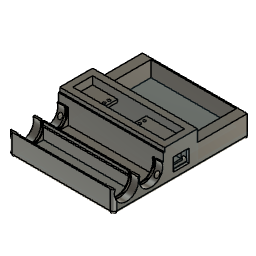
servo holder v10 (Autodesk Fusion 360 design; units mm, degrees)
Autodesk Fusion 360 part; units mm, degrees
sketch "Sketch1" plane through (0, 0, 0) normal (0, 0, 1) x (1, 0, 0)
  line L0 (35, 7.5) -> (-35, 7.5)
  line L1 (-35, 7.5) -> (-35, -7.5)
  line L2 (-35, -7.5) -> (35, -7.5)
  line L3 (35, -7.5) -> (35, 7.5)
  line L4 (35, 7.5) -> (-35, -7.5) construction
  line L5 (-35, 7.5) -> (35, -7.5) construction
  dimension "d1" = 70
  dimension "d2" = 15
  constraint horizontal L0
  constraint perpendicular L0 L1
  constraint parallel L0 L2
  constraint parallel L1 L3
  constraint coincident L4 origin
  constraint coincident L5 origin
  measures "d1" distance of L1.end L2.end
  measures "d2" distance of L0.end L1.end
extrude "Extrude1" add sketch "Sketch1" along normal blind 5
sketch "Sketch2" plane through (0, 0, 5) normal (0, 0, 1) x (-1, 0, 0)
  line L0 (-35, 7.5) -> (-35, -7.5)
  line L1 (-35, -7.5) -> (35, -7.5)
  line L2 (35, -7.5) -> (35, 7.5)
  line L3 (35, 7.5) -> (-35, 7.5)
sketch "Sketch3" plane through (0, 0, 0) normal (0, 0, -1) x (1, 0, 0)
  line L0 (35, -7.5) -> (35, 7.5)
  line L1 (35, 7.5) -> (-35, 7.5)
  line L2 (-35, 7.5) -> (-35, -7.5)
  line L3 (-35, -7.5) -> (35, -7.5)
  line L4 (35, 7.5) -> (40, 7.5)
  line L5 (40, 7.5) -> (40, -7.5)
  line L6 (40, -7.5) -> (35, -7.5)
  line L7 (35, -7.5) -> (35, 7.5)
  line L8 (-35, 7.5) -> (-40, 7.5)
  line L9 (-40, 7.5) -> (-40, -7.5)
  line L10 (-40, -7.5) -> (-35, -7.5)
  line L11 (-35, -7.5) -> (-35, 7.5)
  dimension "d9" = 5
  dimension "d10" = 15
  dimension "d11" = 5
  dimension "d12" = 15
  constraint horizontal L4
  constraint vertical L5
  constraint horizontal L6
  constraint vertical L7
  constraint coincident L0.end L1.start
  constraint horizontal L8
  constraint vertical L9
  constraint horizontal L10
  constraint vertical L11
  constraint coincident L1.end L2.start
  measures "d9" distance of L0.end L4.end
  measures "d10" distance of L0.end L0.start
  measures "d11" distance of L1.end L8.end
  measures "d12" distance of L1.end L2.end
extrude "Extrude2" add sketch "Sketch3" against normal blind 26 contours L0 L4 L5 L6 L7 | L2 L8 L9 L10 L11
sketch "Sketch4" plane through (0, -7.5, 0) normal (0, -1, 0) x (1, 0, 0)
  line L0 (-40, 0) -> (40, 0)
  line L1 (40, 0) -> (40, 26)
  line L2 (40, 26) -> (35, 26)
  line L3 (35, 26) -> (35, 5)
  line L4 (35, 5) -> (-35, 5)
  line L5 (-35, 5) -> (-35, 26)
  line L6 (-35, 26) -> (-40, 26)
  line L7 (-40, 26) -> (-40, 0)
  line L8 (6, 20) -> (35, 20)
  line L9 (35, 20) -> (35, 18)
  line L10 (35, 18) -> (6, 18)
  line L11 (6, 18) -> (6, 20)
  line L12 (-35, 5) -> (35, 5)
  line L13 (-35, 20) -> (-16, 20)
  line L14 (-16, 20) -> (-16, 18)
  line L15 (-16, 18) -> (-35, 18)
  line L16 (-35, 18) -> (-35, 20)
  dimension "d15" = 29
  dimension "d16" = 2
  dimension "d17" = 13
  dimension "d18" = 5
  dimension "d19" = 19
  dimension "d20" = 2
  dimension "d21" = 13
  dimension "d22" = 5
  constraint horizontal L8
  constraint vertical L9
  constraint horizontal L10
  constraint vertical L11
  constraint horizontal L13
  constraint vertical L14
  constraint horizontal L15
  constraint vertical L16
  measures "d15" distance of L8.start L8.end
  measures "d16" distance of L8.start L10.end
  measures "d17" distance of L10 L12
  measures "d18" distance of L1 L9
  measures "d19" distance of L13.start L13.end
  measures "d20" distance of L13.start L15.end
  measures "d21" distance of L12 L15
  measures "d22" distance of L7 L13.start
extrude "Extrude3" add sketch "Sketch4" against normal blind 15 contours L5 L13 L14 L15 L16 | L3 L8 L9 L10 L11
sketch "Sketch5" plane through (0, 0, 20) normal (0, 0, 1) x (-1, 0, 0)
  line L0 (-6, 7.5) -> (-35, 7.5)
  line L1 (-35, 7.5) -> (-35, -7.5)
  line L2 (-35, -7.5) -> (-6, -7.5)
  line L3 (-6, -7.5) -> (-6, 7.5)
  circle A0 centre (-8.54, 3.5) radius 1
  circle A1 centre (-8.54, -3.5) radius 1
  circle A2 centre (-8.54, 0) radius 1
  circle A3 centre (-8.54, 3.5) radius 1
  circle A4 centre (-8.54, 0) radius 1
  circle A5 centre (18.54, 3.5) radius 1
  circle A6 centre (18.54, -3.5) radius 1
  circle A7 centre (18.54, 0) radius 1
  line L4 (16, 7.5) -> (16, -7.5)
  dimension "d25" = 2
  dimension "d36" = 2
  dimension "d44" = 2
  dimension "d45" = 2.54
  dimension "d48" = 3.5
  dimension "d49" = 3.5
  dimension "d50" = 2
  dimension "d53" = 3.5
  dimension "d55" = 2
  dimension "d56" = 2
  dimension "d57" = 2
  dimension "d58" = 3.5
  dimension "d59" = 3.5
  dimension "d60" = 2.54
  measures "d25" diameter of A0
  measures "d36" diameter of A1
  measures "d44" diameter of A2
  measures "d45" distance of L3 A2.centre
  measures "d48" distance of A0.centre A2.centre
  measures "d49" distance of A1.centre A2.centre
  measures "d50" diameter of A3
  measures "d53" distance of A2.centre A0.centre
  measures "d55" diameter of A5
  measures "d56" diameter of A6
  measures "d57" diameter of A7
  measures "d58" distance of A7.centre A5.centre
  measures "d59" distance of A7.centre A6.centre
  measures "d60" distance of A7.centre L4
extrude "Extrude4" cut sketch "Sketch5" against normal blind 2 contours A0 A3 | A1 | A2 A4 | A5 | A6 | A7
sketch "Sketch6" plane through (0, 0, 0) normal (0, 0, -1) x (1, 0, 0)
  line L0 (40, 7.5) -> (-40, 7.5)
  line L1 (-40, 7.5) -> (-40, -7.5)
  line L2 (-40, -7.5) -> (40, -7.5)
  line L3 (40, -7.5) -> (40, 7.5)
  line L4 (-40, 7.5) -> (40, 7.5)
  line L5 (40, 7.5) -> (40, 12.5)
  line L6 (40, 12.5) -> (-40, 12.5)
  line L7 (-40, 12.5) -> (-40, 7.5)
  line L8 (-40, -7.5) -> (40, -7.5)
  line L9 (40, -7.5) -> (40, -12.5)
  line L10 (40, -12.5) -> (-40, -12.5)
  line L11 (-40, -12.5) -> (-40, -7.5)
  dimension "d63" = 80
  dimension "d64" = 5
  dimension "d65" = 80
  dimension "d66" = 5
  constraint horizontal L4
  constraint vertical L5
  constraint horizontal L6
  constraint vertical L7
  constraint coincident L0.end L1.start
  constraint horizontal L8
  constraint vertical L9
  constraint horizontal L10
  constraint vertical L11
  constraint coincident L1.end L2.start
  measures "d63" distance of L0.end L0.start
  measures "d64" distance of L0.end L6.end
  measures "d65" distance of L1.end L2.end
  measures "d66" distance of L1.end L10.end
extrude "Extrude5" add sketch "Sketch6" against normal blind 26 contours L0 L4 L5 L6 L7 | L2 L8 L9 L10 L11
sketch "Sketch7" plane through (0, 0, 5) normal (0, 0, 1) x (1, 0, 0)
  line L0 (-15.5, 7.5) -> (5.5, 7.5)
  line L1 (5.5, 7.5) -> (5.5, 6.1)
  line L2 (5.5, 6.1) -> (-15.5, 6.1)
  line L3 (-15.5, 6.1) -> (-15.5, 7.5)
  line L4 (-15.3542, -7.4527) -> (5.6458, -7.4527)
  line L5 (5.6458, -7.4527) -> (5.6458, -6.0527)
  line L6 (5.6458, -6.0527) -> (-15.3542, -6.0527)
  line L7 (-15.3542, -6.0527) -> (-15.3542, -7.4527)
  dimension "d69" = 21
  dimension "d70" = 1.4
  dimension "d71" = 21
  dimension "d72" = 1.4
  constraint horizontal L0
  constraint vertical L1
  constraint horizontal L2
  constraint vertical L3
  constraint horizontal L4
  constraint vertical L5
  constraint horizontal L6
  constraint vertical L7
  measures "d69" distance of L0.start L0.end
  measures "d70" distance of L0.start L2.end
  measures "d71" distance of L4.start L4.end
  measures "d72" distance of L4.start L6.end
extrude "Extrude6" add sketch "Sketch7" along normal blind 5
sketch "Sketch8" plane through (40, 0, 0) normal (1, 0, 0) x (0, 1, 0)
  line L0 (-12.5, 0) -> (12.5, 0)
  line L1 (12.5, 0) -> (12.5, 26)
  line L2 (12.5, 26) -> (-12.5, 26)
  line L3 (-12.5, 26) -> (-12.5, 0)
  line L4 (-5, 15.5) -> (5, 15.5)
  line L5 (5, 15.5) -> (5, 7.5)
  line L6 (5, 7.5) -> (-5, 7.5)
  line L7 (-5, 7.5) -> (-5, 15.5)
  dimension "d75" = 10
  dimension "d76" = 8
  dimension "d77" = 7.5
  dimension "d78" = 7.5
  constraint horizontal L4
  constraint vertical L5
  constraint horizontal L6
  constraint vertical L7
  measures "d75" distance of L4.start L4.end
  measures "d76" distance of L4.start L6.end
  measures "d77" distance of L1 L5
  measures "d78" distance of L0 L6
extrude "Extrude7" cut sketch "Sketch8" against normal blind 5 contours L4 L5 L6 L7
sketch "Sketch9" plane through (0, 0, 0) normal (0, 0, -1) x (1, 0, 0)
  line L0 (-40, 12.5) -> (-40, -12.5)
  line L1 (-40, -12.5) -> (40, -12.5)
  line L2 (40, -12.5) -> (40, 12.5)
  line L3 (40, 12.5) -> (-40, 12.5)
  line L4 (-40, 12.5) -> (40, 12.5)
  line L5 (40, 12.5) -> (40, 32.5)
  line L6 (40, 32.5) -> (-40, 32.5)
  line L7 (-40, 32.5) -> (-40, 12.5)
  dimension "d81" = 80
  dimension "d82" = 20
  constraint horizontal L4
  constraint vertical L5
  constraint horizontal L6
  constraint vertical L7
  constraint coincident L0.start L3.end
  measures "d81" distance of L0.start L2.end
  measures "d82" distance of L0.start L6.end
extrude "Extrude8" add sketch "Sketch9" against normal blind 5 contours L3 L4 L5 L6 L7
sketch "Sketch10" plane through (0, 0, 5) normal (0, 0, 1) x (-1, 0, 0)
  line L0 (40, 12.5) -> (40, 32.5)
  line L1 (40, 32.5) -> (-40, 32.5)
  line L2 (-40, 32.5) -> (-40, 12.5)
  line L3 (-40, 12.5) -> (40, 12.5)
  line L4 (40, 12.5) -> (-40, 12.5)
  line L5 (-40, 12.5) -> (-40, 13.5)
  line L6 (-40, 13.5) -> (40, 13.5)
  line L7 (40, 13.5) -> (40, 12.5)
  dimension "d85" = 80
  dimension "d86" = 1
  constraint horizontal L4
  constraint vertical L5
  constraint horizontal L6
  constraint vertical L7
  constraint coincident L0.start L3.end
  measures "d85" distance of L0.start L2.end
  measures "d86" distance of L0.start L6.end
extrude "Extrude9" add sketch "Sketch10" along normal blind 18 contours L0 L2 L3 L4 L5 L6 L7
sketch "Sketch11" plane through (0, 0, 5) normal (0, 0, 1) x (-1, 0, 0)
  line L0 (-40, 13.5) -> (40, 13.5)
  line L1 (40, 13.5) -> (40, 32.5)
  line L2 (40, 32.5) -> (-40, 32.5)
  line L3 (-40, 32.5) -> (-40, 13.5)
  line L4 (-40, 13.5) -> (-33.5, 13.5)
  line L5 (-33.5, 13.5) -> (-33.5, 32.5)
  line L6 (-33.5, 32.5) -> (-40, 32.5)
  line L7 (-40, 32.5) -> (-40, 13.5)
  line L8 (40, 13.5) -> (33.5, 13.5)
  line L9 (33.5, 13.5) -> (33.5, 32.5)
  line L10 (33.5, 32.5) -> (40, 32.5)
  line L11 (40, 32.5) -> (40, 13.5)
  dimension "d89" = 6.5
  dimension "d90" = 6.5
  constraint horizontal L4
  constraint vertical L5
  constraint horizontal L6
  constraint vertical L7
  constraint coincident L0.start L3.end
  constraint horizontal L8
  constraint vertical L9
  constraint horizontal L10
  constraint vertical L11
  constraint coincident L0.end L1.start
  measures "d89" distance of L0.start L4.end
  measures "d90" distance of L0.end L8.end
extrude "Extrude10" add sketch "Sketch11" along normal blind 12 contours L0 L2 L3 L4 L5 L6 L7 | L0 L1 L2 L8 L9 L10 L11
sketch "Sketch12" plane through (40, 0, 0) normal (1, 0, 0) x (0, 1, 0)
  line L0 (5, 15.5) -> (5, 7.5)
  line L1 (5, 7.5) -> (-5, 7.5)
  line L2 (-5, 7.5) -> (-5, 15.5)
  line L3 (-5, 15.5) -> (5, 15.5)
  line L4 (-32.5, 0) -> (12.5, 0)
  line L5 (12.5, 0) -> (12.5, 26)
  line L6 (12.5, 26) -> (-12.5, 26)
  line L7 (-12.5, 26) -> (-12.5, 23)
  line L8 (-12.5, 23) -> (-13.5, 23)
  line L9 (-13.5, 23) -> (-13.5, 17)
  line L10 (-13.5, 17) -> (-32.5, 17)
  line L11 (-32.5, 17) -> (-32.5, 0)
  circle A0 centre (-23, 14) radius 9
  dimension "d93" = 18
  dimension "d94" = 14
  dimension "d95" = 9.5
  measures "d93" diameter of A0
  measures "d94" distance of L4 A0.centre
  measures "d95" distance of L11 A0.centre
extrude "Extrude11" cut sketch "Sketch12" against normal blind 80 contours L10 A0 | L10 A0
sketch "Sketch13" plane through (0, 0, 5) normal (0, 0, 1) x (-1, 0, 0)
  line L0 (33.5, 23) -> (33.5, 32.5)
  line L1 (33.5, 32.5) -> (-33.5, 32.5)
  line L2 (-33.5, 32.5) -> (-33.5, 23)
  line L3 (-33.5, 23) -> (-33.5, 13.5)
  line L4 (-33.5, 13.5) -> (33.5, 13.5)
  line L5 (33.5, 13.5) -> (33.5, 23)
  line L6 (33.5, 13.5) -> (32.5, 13.5)
  line L7 (32.5, 13.5) -> (32.5, 32.5)
  line L8 (32.5, 32.5) -> (33.5, 32.5)
  line L9 (33.5, 32.5) -> (33.5, 13.5)
  line L10 (-33.5, 13.5) -> (-32.5, 13.5)
  line L11 (-32.5, 13.5) -> (-32.5, 32.5)
  line L12 (-32.5, 32.5) -> (-33.5, 32.5)
  line L13 (-33.5, 32.5) -> (-33.5, 13.5)
  dimension "d98" = 1
  dimension "d99" = 1
  constraint horizontal L6
  constraint vertical L7
  constraint horizontal L8
  constraint vertical L9
  constraint coincident L4.end L5.start
  constraint horizontal L10
  constraint vertical L11
  constraint horizontal L12
  constraint vertical L13
  constraint coincident L3.end L4.start
  measures "d98" distance of L4.end L6.end
  measures "d99" distance of L3.end L10.end
extrude "Extrude12" add sketch "Sketch13" along normal blind 12 contours L0 L1 L4 L5 L6 L7 L8 L9 | L1 L2 L3 L4 L10 L11 L12 L13
delete_face "DeleteFace1" 1 faces at (33.5, -20.1151, 14.4205)
delete_face "DeleteFace2" 1 faces at (-33.5, -25.1677, 12.4715)
sketch "Sketch14" plane through (0, 0, 5) normal (0, 0, 1) x (-1, 0, 0)
  line L0 (-32.5, 23) -> (-32.5, 13.5)
  line L1 (-32.5, 13.5) -> (32.5, 13.5)
  line L2 (32.5, 13.5) -> (32.5, 23)
  line L3 (32.5, 23) -> (32.5, 32.5)
  line L4 (32.5, 32.5) -> (-32.5, 32.5)
  line L5 (-32.5, 32.5) -> (-32.5, 23)
  line L6 (-33, 13.5) -> (-34.5, 13.5)
  line L7 (-34.5, 13.5) -> (-34.5, 32.5)
  line L8 (-34.5, 32.5) -> (-33, 32.5)
  line L9 (-33, 32.5) -> (-33, 13.5)
  dimension "d102" = 1.5
  dimension "d103" = 19
  dimension "d104" = 0.5
  constraint horizontal L6
  constraint vertical L7
  constraint horizontal L8
  constraint vertical L9
  measures "d102" distance of L6.start L6.end
  measures "d103" distance of L6.start L8.end
  measures "d104" distance of L0 L9
extrude "Extrude13" cut sketch "Sketch14" along normal blind 12 contours L6 L7 L8 L9
sketch "Sketch15" plane through (0, 0, 5) normal (0, 0, 1) x (-1, 0, 0)
  line L0 (-32.5, 23) -> (-32.5, 13.5)
  line L1 (-32.5, 13.5) -> (32.5, 13.5)
  line L2 (32.5, 13.5) -> (32.5, 23)
  line L3 (32.5, 23) -> (32.5, 32.5)
  line L4 (32.5, 32.5) -> (-32.5, 32.5)
  line L5 (-32.5, 32.5) -> (-32.5, 23)
  line L6 (34.5, 13.5004) -> (33, 13.5004)
  line L7 (33, 13.5004) -> (33, 32.5004)
  line L8 (33, 32.5004) -> (34.5, 32.5004)
  line L9 (34.5, 32.5004) -> (34.5, 13.5004)
  dimension "d107" = 1.5
  dimension "d108" = 19
  dimension "d109" = 0.5
  constraint horizontal L6
  constraint vertical L7
  constraint horizontal L8
  constraint vertical L9
  measures "d107" distance of L6.start L6.end
  measures "d108" distance of L6.start L8.end
  measures "d109" distance of L2 L7
extrude "Extrude14" cut sketch "Sketch15" along normal blind 12 contours L6 L7 L8 L9
sketch "Sketch16" plane through (0, 0, 0) normal (0, 0, -1) x (1, 0, 0)
  line L0 (-40, 32.5) -> (-40, -12.5)
  line L1 (-40, -12.5) -> (40, -12.5)
  line L2 (40, -12.5) -> (40, 32.5)
  line L3 (40, 32.5) -> (-40, 32.5)
  line L4 (-40, 32.5) -> (40, 32.5)
  line L5 (40, 32.5) -> (40, 51.5)
  line L6 (40, 51.5) -> (-40, 51.5)
  line L7 (-40, 51.5) -> (-40, 32.5)
  line L8 (40, -12.5) -> (-40, -12.5)
  line L9 (-40, -12.5) -> (-40, -50.5)
  line L10 (-40, -50.5) -> (40, -50.5)
  line L11 (40, -50.5) -> (40, -12.5)
  dimension "d112" = 80
  dimension "d113" = 19
  dimension "d114" = 80
  dimension "d115" = 38
  constraint horizontal L4
  constraint vertical L5
  constraint horizontal L6
  constraint vertical L7
  constraint coincident L0.start L3.end
  constraint horizontal L8
  constraint vertical L9
  constraint horizontal L10
  constraint vertical L11
  constraint coincident L1.end L2.start
  measures "d112" distance of L0.start L2.end
  measures "d113" distance of L0.start L6.end
  measures "d114" distance of L1.end L0.end
  measures "d115" distance of L1.end L10.end
extrude "Extrude15" add sketch "Sketch16" against normal blind 5 contours L3 L4 L5 L6 L7 | L1 L8 L9 L10 L11
sketch "Sketch17" plane through (0, 0, 5) normal (0, 0, 1) x (-1, 0, 0)
  line L0 (33, 32.5) -> (33, 23)
  line L1 (33, 23) -> (33, 13.5004)
  line L2 (33, 13.5004) -> (34.5, 13.5004)
  line L3 (34.5, 13.5004) -> (34.5, 23)
  line L4 (34.5, 23) -> (34.5, 32.5)
  line L5 (34.5, 32.5) -> (40, 32.5)
  line L6 (40, 32.5) -> (40, 51.5)
  line L7 (40, 51.5) -> (-40, 51.5)
  line L8 (-40, 51.5) -> (-40, 32.5)
  line L9 (-40, 32.5) -> (-34.5, 32.5)
  line L10 (-34.5, 32.5) -> (-34.5, 23)
  line L11 (-34.5, 23) -> (-34.5, 13.5)
  line L12 (-34.5, 13.5) -> (-33, 13.5)
  line L13 (-33, 13.5) -> (-33, 23)
  line L14 (-33, 23) -> (-33, 32.5)
  line L15 (-33, 32.5) -> (-32.5, 32.5)
  line L16 (-32.5, 32.5) -> (-32.5, 23)
  line L17 (-32.5, 23) -> (-32.5, 13.5)
  line L18 (-32.5, 13.5) -> (32.5, 13.5)
  line L19 (32.5, 13.5) -> (32.5, 23)
  line L20 (32.5, 23) -> (32.5, 32.5)
  line L21 (32.5, 32.5) -> (33, 32.5)
  line L22 (40, 32.5) -> (32.5, 32.5)
  line L23 (32.5, 32.5) -> (32.5, 51.5)
  line L24 (32.5, 51.5) -> (40, 51.5)
  line L25 (40, 51.5) -> (40, 32.5)
  line L26 (-40, 32.5) -> (-32.5, 32.5)
  line L27 (-32.5, 32.5) -> (-32.5, 51.5)
  line L28 (-32.5, 51.5) -> (-40, 51.5)
  line L29 (-40, 51.5) -> (-40, 32.5)
  dimension "d118" = 7.5
  dimension "d119" = 19
  dimension "d120" = 7.5
  dimension "d121" = 19
  constraint horizontal L22
  constraint vertical L23
  constraint horizontal L24
  constraint vertical L25
  constraint coincident L5.end L6.start
  constraint horizontal L26
  constraint vertical L27
  constraint horizontal L28
  constraint vertical L29
  constraint coincident L8.end L9.start
  measures "d118" distance of L5.end L20.end
  measures "d119" distance of L5.end L6.end
  measures "d120" distance of L8.end L15.end
  measures "d121" distance of L8.end L7.end
extrude "Extrude16" add sketch "Sketch17" along normal blind 12 contours L5 L6 L7 L21 L22 L23 L24 L25 | L7 L8 L9 L15 L26 L27 L28 L29
sketch "Sketch18" plane through (0, 0, 5) normal (0, 0, 1) x (-1, 0, 0)
  line L0 (32.5, 23) -> (32.5, 51.5)
  line L1 (32.5, 51.5) -> (-32.5, 51.5)
  line L2 (-32.5, 51.5) -> (-32.5, 23)
  line L3 (-32.5, 23) -> (-32.5, 13.5)
  line L4 (-32.5, 13.5) -> (32.5, 13.5)
  line L5 (32.5, 13.5) -> (32.5, 23)
  line L6 (-32.5, 31.5206) -> (32.5, 31.5206)
  line L7 (32.5, 31.5206) -> (32.5, 32.5206)
  line L8 (32.5, 32.5206) -> (-32.5, 32.5206)
  line L9 (-32.5, 32.5206) -> (-32.5, 31.5206)
  dimension "d124" = 1
  constraint horizontal L6
  constraint vertical L7
  constraint horizontal L8
  constraint vertical L9
  constraint coincident L2 L6.start
  measures "d124" distance of L6.start L8.end
extrude "Extrude17" add sketch "Sketch18" along normal blind 12 contours L0 L2 L6 L7 L8 L9
sketch "Sketch19" plane through (0, 0, 5) normal (0, 0, 1) x (-1, 0, 0)
  line L0 (-32.5, 32.5206) -> (32.5, 32.5206)
  line L1 (32.5, 32.5206) -> (32.5, 51.5)
  line L2 (32.5, 51.5) -> (-32.5, 51.5)
  line L3 (-32.5, 51.5) -> (-32.5, 32.5206)
sketch "Sketch21" plane through (0, 0, 17) normal (0, 0, 1) x (-1, 0, 0)
  line L0 (33, 31.4853) -> (33, 32.5)
  line L1 (33, 32.5) -> (34.5, 32.5)
  line L2 (34.5, 32.5) -> (34.5, 31.4853)
  line L3 (34.5, 31.4853) -> (40, 31.4853)
  line L4 (40, 31.4853) -> (40, 51.5)
  line L5 (40, 51.5) -> (32.5, 51.5)
  line L6 (32.5, 51.5) -> (32.5, 32.5206)
  line L7 (32.5, 32.5206) -> (-32.5, 32.5206)
  line L8 (-32.5, 32.5206) -> (-32.5, 51.5)
  line L9 (-32.5, 51.5) -> (-40, 51.5)
  line L10 (-40, 51.5) -> (-40, 31.4853)
  line L11 (-40, 31.4853) -> (-34.5, 31.4853)
  line L12 (-34.5, 31.4853) -> (-34.5, 32.5)
  line L13 (-34.5, 32.5) -> (-33, 32.5)
  line L14 (-33, 32.5) -> (-33, 31.4853)
  line L15 (-33, 31.4853) -> (-32.5, 31.4853)
  line L16 (-32.5, 31.4853) -> (-32.5, 31.5206)
  line L17 (-32.5, 31.5206) -> (32.5, 31.5206)
  line L18 (32.5, 31.5206) -> (32.5, 31.4853)
  line L19 (32.5, 31.4853) -> (33, 31.4853)
  line L20 (34.5, 32.5) -> (33, 32.5)
  line L21 (33, 32.5) -> (33, 50.5)
  line L22 (33, 50.5) -> (34.5, 50.5)
  line L23 (34.5, 50.5) -> (34.5, 32.5)
  line L24 (-34.5, 32.5) -> (-33, 32.5)
  line L25 (-33, 32.5) -> (-33, 50.5)
  line L26 (-33, 50.5) -> (-34.5, 50.5)
  line L27 (-34.5, 50.5) -> (-34.5, 32.5)
  line L28 (32.5, 51.5) -> (-32.5, 51.5)
  line L29 (-32.5, 51.5) -> (-32.5, 50.5)
  line L30 (-32.5, 50.5) -> (32.5, 50.5)
  line L31 (32.5, 50.5) -> (32.5, 51.5)
  dimension "d129" = 1.5
  dimension "d130" = 18
  dimension "d131" = 1.5
  dimension "d132" = 18
  dimension "d133" = 65
  dimension "d134" = 1
  constraint horizontal L20
  constraint vertical L21
  constraint horizontal L22
  constraint vertical L23
  constraint coincident L1.end L2.start
  constraint horizontal L24
  constraint vertical L25
  constraint horizontal L26
  constraint vertical L27
  constraint coincident L12.end L13.start
  constraint horizontal L28
  constraint vertical L29
  constraint horizontal L30
  constraint vertical L31
  constraint coincident L5.end L6.start
  measures "d129" distance of L1.end L0.end
  measures "d130" distance of L1.end L22.end
  measures "d131" distance of L12.end L13.end
  measures "d132" distance of L12.end L26.end
  measures "d133" distance of L5.end L8.end
  measures "d134" distance of L5.end L30.end
extrude "Extrude18" cut sketch "Sketch21" against normal blind 12 contours L1 L20 L21 L22 L23 | L13 L24 L25 L26 L27
sketch "Sketch22" plane through (0, 0, 5) normal (0, 0, 1) x (1, 0, 0)
sketch "Sketch23" plane through (0, 0, 5) normal (0, 0, 1) x (1, 0, 0)
sketch "Sketch24" plane through (32.5, 0, 0) normal (-1, 0, 0) x (0, -1, 0)
  line L0 (32.5206, 17) -> (32.5206, 5)
  line L1 (32.5206, 5) -> (51.5, 5)
  line L2 (51.5, 5) -> (51.5, 17)
  line L3 (51.5, 17) -> (32.5206, 17)
  line L4 (51.5, 17) -> (50.5, 17)
  line L5 (50.5, 17) -> (50.5, 5)
  line L6 (50.5, 5) -> (51.5, 5)
  line L7 (51.5, 5) -> (51.5, 17)
  dimension "d137" = 1
  dimension "d138" = 12
  constraint horizontal L4
  constraint vertical L5
  constraint horizontal L6
  constraint vertical L7
  constraint coincident L2.end L3.start
  measures "d137" distance of L2.end L4.end
  measures "d138" distance of L2.end L1.end
extrude "Extrude19" add sketch "Sketch24" along normal blind 65 contours L1 L2 L3 L4 L5 L6 L7
sketch "Sketch25" plane through (40, 0, 0) normal (1, 0, 0) x (0, 1, 0)
  arc A0 (-31.4853, 17) -> (-14.5147, 17) centre (-23, 14) ccw
  line L0 (-31.4853, 17) -> (-51.5, 17)
  line L1 (-51.5, 17) -> (-51.5, 0)
  line L2 (-51.5, 0) -> (50.5, 0)
  line L3 (50.5, 0) -> (50.5, 5)
  line L4 (50.5, 5) -> (12.5, 5)
  line L5 (12.5, 5) -> (12.5, 26)
  line L6 (12.5, 26) -> (-12.5, 26)
  line L7 (-12.5, 26) -> (-12.5, 23)
  line L8 (-12.5, 23) -> (-13.5, 23)
  line L9 (-13.5, 23) -> (-13.5, 17)
  line L10 (-13.5, 17) -> (-14.5147, 17)
  line L11 (5, 15.5) -> (5, 7.5)
  line L12 (5, 7.5) -> (-5, 7.5)
  line L13 (-5, 7.5) -> (-5, 15.5)
  line L14 (-5, 15.5) -> (5, 15.5)
  circle A1 centre (-41.5, 14) radius 9
  dimension "d141" = 18
  dimension "d142" = 14
  dimension "d143" = 10
  measures "d141" diameter of A1
  measures "d142" distance of L2 A1.centre
  measures "d143" distance of L1 A1.centre
extrude "Extrude20" cut sketch "Sketch25" against normal blind 80 contours L0 A1 | L0 A1
fillet "Fillet1" radius 2.5 1 edges at (0, -51.5, 0)
fillet "Fillet2" radius 2.5 3 edges at (-40, 0.75, 0) (-40, -50.7678, 0.7322) (-40, -51.5, 9.75)
fillet "Fillet3" radius 2.5 3 edges at (40, 0.75, 0) (40, -50.7678, 0.7322) (40, -51.5, 9.75)
sketch "Sketch27" plane through (0, 12.5, 0) normal (0, 1, 0) x (-1, 0, 0)
  line L0 (-40, 5) -> (40, 5)
  line L1 (40, 5) -> (40, 26)
  line L2 (40, 26) -> (-40, 26)
  line L3 (-40, 26) -> (-40, 5)
  circle A0 centre (37, 9.75) radius 1.75
  dimension "d155" = 3.5
  dimension "d156" = 3
  dimension "d157" = 4.75
  measures "d155" diameter of A0
  measures "d156" distance of L1 A0.centre
  measures "d157" distance of L0 A0.centre
extrude "Extrude21" cut sketch "Sketch27" along normal blind -30 and the other way blind -10 contours A0
sketch "Sketch28" plane through (0, 12.5, 0) normal (0, 1, 0) x (-1, 0, 0)
  circle A0 centre (37, 9.75) radius 1.75
  line L0 (-40, 5) -> (40, 5)
  line L1 (40, 5) -> (40, 26)
  line L2 (40, 26) -> (-40, 26)
  line L3 (-40, 26) -> (-40, 5)
  circle A1 centre (-37.5, 8.75) radius 1.75
  dimension "d162" = 3.5
  dimension "d163" = 2.5
  dimension "d164" = 3.75
  measures "d162" diameter of A1
  measures "d163" distance of L3 A1.centre
  measures "d164" distance of L0 A1.centre
extrude "Extrude22" cut sketch "Sketch28" against normal blind 30 contours A1
sketch "Sketch29" plane through (40, 0, 0) normal (1, 0, 0) x (0, 1, 0)
  line L0 (-49, 2.5) -> (50.5, 2.5)
  line L1 (50.5, 2.5) -> (50.5, 5)
  line L2 (50.5, 5) -> (12.5, 5)
  line L3 (12.5, 5) -> (12.5, 26)
  line L4 (12.5, 26) -> (-12.5, 26)
  line L5 (-12.5, 26) -> (-12.5, 23)
  line L6 (-12.5, 23) -> (-13.5, 23)
  line L7 (-13.5, 23) -> (-13.5, 17)
  line L8 (-13.5, 17) -> (-14.5147, 17)
  arc A0 (-31.4853, 17) -> (-14.5147, 17) centre (-23, 14) ccw
  line L9 (-31.4853, 17) -> (-33.0147, 17)
  arc A1 (-49, 9.0251) -> (-33.0147, 17) centre (-41.5, 14) ccw
  line L10 (-49, 9.0251) -> (-49, 2.5)
  line L11 (5, 15.5) -> (5, 7.5)
  line L12 (5, 7.5) -> (-5, 7.5)
  line L13 (-5, 7.5) -> (-5, 15.5)
  line L14 (-5, 15.5) -> (5, 15.5)
fillet "Fillet4" radius 1 4 edges at (40, 0, 7.5) (40, 5, 11.5) (40, 0, 15.5) (40, -5, 11.5)
sketch "Sketch30" plane through (0, 0, 5) normal (0, 0, 1) x (-1, 0, 0)
  line L0 (-40, -12.5) -> (-40, -50.5)
  line L1 (-40, -50.5) -> (40, -50.5)
  line L2 (40, -50.5) -> (40, -12.5)
  line L3 (40, -12.5) -> (-40, -12.5)
  line L4 (40, -50.5) -> (32.5, -50.5)
  line L5 (32.5, -50.5) -> (32.5, -12.5)
  line L6 (32.5, -12.5) -> (40, -12.5)
  line L7 (40, -12.5) -> (40, -50.5)
  line L8 (-40, -50.5) -> (-32.5, -50.5)
  line L9 (-32.5, -50.5) -> (-32.5, -12.5)
  line L10 (-32.5, -12.5) -> (-40, -12.5)
  line L11 (-40, -12.5) -> (-40, -50.5)
  line L12 (32.5, -50.5) -> (-32.5, -50.5)
  line L13 (-32.5, -50.5) -> (-32.5, -49.5)
  line L14 (-32.5, -49.5) -> (32.5, -49.5)
  line L15 (32.5, -49.5) -> (32.5, -50.5)
  dimension "d169" = 7.5
  dimension "d170" = 38
  dimension "d171" = 7.5
  dimension "d172" = 38
  dimension "d173" = 65
  dimension "d174" = 1
  constraint horizontal L4
  constraint vertical L5
  constraint horizontal L6
  constraint vertical L7
  constraint coincident L1.end L2.start
  constraint horizontal L8
  constraint vertical L9
  constraint horizontal L10
  constraint vertical L11
  constraint coincident L0.end L1.start
  constraint horizontal L12
  constraint vertical L13
  constraint horizontal L14
  constraint vertical L15
  measures "d169" distance of L1.end L4.end
  measures "d170" distance of L1.end L2.end
  measures "d171" distance of L0.end L8.end
  measures "d172" distance of L0.end L0.start
  measures "d173" distance of L4.end L8.end
  measures "d174" distance of L4.end L14.end
extrude "Extrude23" add sketch "Sketch30" along normal blind 12 contours L0 L1 L3 L8 L9 L10 L11 L13 | L1 L5 L9 L12 L13 L14 L15 | L1 L2 L3 L4 L5 L6 L7 L15
sketch "Sketch31" plane through (0, 0, 5) normal (0, 0, 1) x (-1, 0, 0)
  line L0 (32.5, -49.5) -> (32.5, -12.5)
  line L1 (32.5, -12.5) -> (-32.5, -12.5)
  line L2 (-32.5, -12.5) -> (-32.5, -49.5)
  line L3 (-32.5, -49.5) -> (32.5, -49.5)
equation "d94 = 9 mm + 5 mm"
equation "d95 = 9 mm + 0.5 mm"
equation "d142 = 9 mm + 5 mm"
equation "d143 = 9 mm + 1 mm"
equation "d157 = 1.75 mm + 3 mm"
equation "d164 = 1.75 mm + 2 mm"
